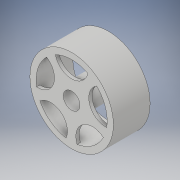
# Autodesk Inventor part: wheeel
Saved by Autodesk Inventor 2019 (Build 230136000, 136)
## iProperties
Created: 2020-02-16
Part Number: wheeel
Material: Generic
Document SubType Name: Modeling
Designer: Hp
Density: 1 g/cm^3
Appearance: Default
Author: Hp
Autodesk Inventor part; units mm, degrees
ref_plane "YZ Plane" through (0, 0, 0) normal (1, 0, 0) x (0, 1, 0)
ref_plane "XZ Plane" through (0, 0, 0) normal (0, 1, 0) x (-1, 0, 0)
ref_plane "XY Plane" through (0, 0, 0) normal (0, 0, 1) x (1, 0, 0)
sketch "Sketch1" plane through (0, 0, 0) normal (0, 0, 1) x (1, 0, 0)
  circle A0 centre (0, 0) radius 25
  circle A1 centre (0, 0) radius 21.3012
  circle A2 centre (0, 0) radius 5
  circle A3 centre (0, 0) radius 7.8951
  dimension "d0" = 50
  dimension "d1" = 10
  constraints: 4 centre point, 2 coincident
  measures "d0" diameter of A0
  measures "d1" diameter of A2
extrude "Extrusion1" add sketch "Sketch1" along normal blind 20
sketch "Sketch2" plane through (0, 0, 20) normal (0, 0, 1) x (1, 0, 0)
  circle A0 centre (0, 0) radius 21.3012 projected
  circle A1 centre (0, 0) radius 25 projected
  circle A2 centre (0, 0) radius 5 projected
  circle A3 centre (0, 0) radius 7.8951 projected
  circle A4 centre (0, 0) radius 5 projected
  circle A5 centre (0, 0) radius 7.8951 projected
extrude "Extrusion2" add sketch "Sketch2" along normal blind 2 contours A0 | A1 | A3
sketch "Sketch3" plane through (0, 0, 22) normal (0, 0, 1) x (1, 0, 0)
  circle A0 centre (0, 0) radius 21.3012 projected
  arc A1 (-9.7206, 18.9539) -> (9.7206, 18.9539) centre (0, 21.3012) ccw
  dimension "d6" = 20
  constraints: 5 point on circle, 1 centre point
  measures "d6" diameter of A1
extrude "Extrusion3" cut sketch "Sketch3" against normal blind 2 contours A1 A0 picked at (2.8527, 17.9876)
pattern_circular "Circular Pattern1" count 5 over 360 about axis through (0, 0, 0) along (0, 0, 1) of "Extrusion3"
body "Solid1"
